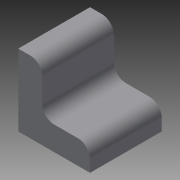
# Autodesk Inventor part: Part
Saved by Autodesk Inventor 2015 (Build 190159000, 159)
## iProperties
Created: 2015-01-15
Part Number: Part
Material: Generic
Document SubType Name: Modeling
Designer: PLTW-Stu-02
Density: 1 g/cm^3
Appearance: Default
Author: PLTW-Stu-02
Autodesk Inventor part; units mm, degrees
ref_plane "YZ Plane" through (0, 0, 0) normal (1, 0, 0) x (0, 1, 0)
ref_plane "XZ Plane" through (0, 0, 0) normal (0, 1, 0) x (-1, 0, 0)
ref_plane "XY Plane" through (0, 0, 0) normal (0, 0, 1) x (1, 0, 0)
sketch "Sketch1" plane through (0, 0, 0) normal (0, 0, 1) x (1, 0, 0)
  line L0 (2.3532, 14.024) -> (40.4532, 14.024)
  line L1 (40.4532, 14.024) -> (40.4532, -24.076)
  line L2 (40.4532, -24.076) -> (2.3532, -24.076)
  line L3 (2.3532, -24.076) -> (2.3532, 14.024)
  point P0 (0, 0)
  dimension "d0" = 38.1
  dimension "d1" = 38.1
  constraints: 8 end point, 2 parallel, 1 horizontal, 1 perpendicular
  measures "d0" distance of L1.end L2.end
  measures "d1" distance of L0.end L1.end
extrude "Extrusion1" add sketch "Sketch1" along normal blind 38.1
sketch "Sketch2" plane through (0, 0, 38.1) normal (0, 0, 1) x (1, 0, 0)
  line L0 (15.0532, 14.024) -> (15.0532, 1.324)
  line L1 (40.4532, 14.024) -> (15.0532, 14.024)
  line L2 (15.0532, 14.024) -> (15.0532, -11.376)
  line L3 (15.0532, -11.376) -> (40.4532, -11.376)
  line L4 (40.4532, -11.376) -> (40.4532, 14.024)
  point P0 (0, 0)
  point P1 (2.3532, 14.024)
  point P2 (40.4532, -24.076)
  dimension "d5" = 12.7
  constraints: 10 end point, 2 parallel, 1 horizontal, 1 perpendicular
  measures "d5" distance of L0.start L0.end
extrude "Extrusion2" cut sketch "Sketch2" against normal through all
fillet "Fillet1" radius 6.35 1 edges at (15.0532, 14.024, 19.05)
fillet "Fillet2" radius 6.35 1 edges at (40.4532, -11.376, 19.05)
fillet "Fillet3" radius 6.35 1 edges at (15.0532, -11.376, 19.05)
body "Solid1"
